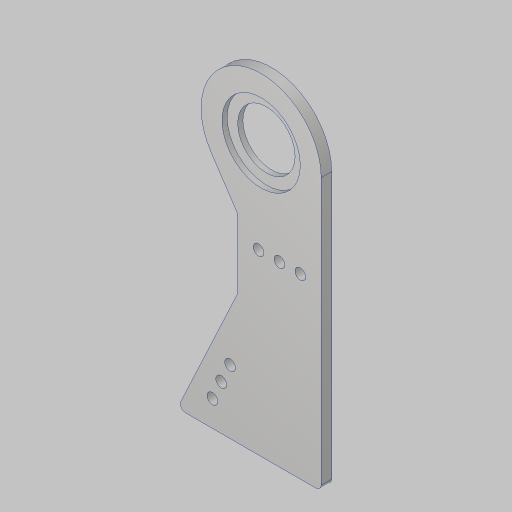
# Autodesk Inventor part: CL7-007
Saved by Autodesk Inventor 2023.5 (Build 275446000, 446)
## iProperties
Created: 2025-03-17
Part Number: CL7-007
Material: Aluminum 6061
Document SubType Name: Modeling
Designer: brand
Density: 2.7 g/cm^3
Appearance: Aluminum - Flat
Author: brand
Autodesk Inventor part; units mm, degrees
ref_plane "YZ Plane" through (0, 0, 0) normal (1, 0, 0) x (0, 1, 0)
ref_plane "XZ Plane" through (0, 0, 0) normal (0, 1, 0) x (-1, 0, 0)
ref_plane "XY Plane" through (0, 0, 0) normal (0, 0, 1) x (1, 0, 0)
sketch "Sketch1" plane through (0, 0, 0) normal (0, 0, 1) x (1, 0, 0)
  circle A0 centre (0, 0) radius 23.8125
  circle A1 centre (0, 0) radius 36.5125
  line L0 (36.5125, -165.1) -> (-14.2875, -165.1) construction
  line L1 (36.5125, 0) -> (36.5125, -165.1)
  line L2 (-36.1762, -4.9442) -> (-14.2875, -165.1) construction
  line L3 (36.5125, -44.45) -> (-14.2875, -44.45) construction
  line L4 (-14.2875, -44.45) -> (-14.2875, -431.8) construction
  line L5 (-14.2875, -431.8) -> (36.5125, -431.8) construction
  line L6 (36.5125, -431.8) -> (36.5125, -44.45) construction
  line L7 (8.7327, -97.2312) -> (-152.2848, -442.5345) construction
  line L8 (-152.2848, -442.5345) -> (-175.3051, -431.8) construction
  line L9 (-175.3051, -431.8) -> (-14.2875, -86.4967) construction
  line L10 (-14.2875, -86.4967) -> (8.7327, -97.2312) construction
  line L11 (36.5125, -431.8) -> (11.1125, -431.8) construction
  line L12 (11.1125, -431.8) -> (11.1125, -501.65) construction
  line L13 (11.1125, -501.65) -> (36.5125, -501.65) construction
  line L14 (36.5125, -501.65) -> (36.5125, -431.8) construction
  line L15 (-150.8125, -431.8) -> (-150.8125, -501.65) construction
  line L16 (-2.7774, -91.864) -> (-19.4192, -127.5524) construction
  line L17 (-36.3765, 3.1489) -> (-36.3765, -165.1) construction
  line L18 (-50.9408, -165.1) -> (36.5125, -165.1)
  line L19 (-50.9408, -165.1) -> (-36.3765, 3.1489)
  line L20 (-50.9408, -165.1) -> (-14.2875, -86.4967)
  line L21 (-14.2875, -44.45) -> (-14.2875, -86.4967)
  line L22 (-14.2875, -44.45) -> (-30.4024, -20.2202)
  point P0 (23.8125, -431.8)
  point P1 (-8.1446, -103.3741)
  point P2 (23.8125, -57.15)
  point P3 (11.1125, -57.15)
  point P4 (-1.5875, -57.15)
  point P5 (11.1125, -44.45)
  point P6 (-13.5119, -114.8842)
  point P7 (-18.8791, -126.3943)
  point P8 (-24.2464, -137.9044)
  point P9 (-29.6137, -149.4145)
  dimension "d0" = 47.625
  dimension "d1" = 12.7
  dimension "d2" = 50.8
  dimension "d3" = 165.1
  dimension "d4" = 50.8
  dimension "d5" = 387.35
  dimension "d6" = 25.4
  dimension "d7" = 25
  dimension "d8" = 381
  dimension "d10" = 25.4
  dimension "d11" = 69.85
  dimension "d13" = 431.8
  dimension "d15" = 187.325
  dimension "d17" = 12.7
  dimension "d18" = 12.7
  dimension "d19" = 12.7
  dimension "d20" = 12.7
  dimension "d23" = 12.7
  constraints: 46 end point, 6 horizontal alignment, 6 parallel, 6 point on line, 5 perpendicular, 4 tangent, 3 collinear, 3 horizontal, 3 midpoint, 3 point on circle, 2 centre point, 2 vertical, 1 coincident, 1 vertical alignment, 5 other
  measures "d0" diameter of A0
  measures "d1" radial gap between concentric circles of A0 A1
  measures "d2" distance of L0.start L0.end
  measures "d3" distance from line of L0 point (0, 0)
  measures "d4" distance of L5.end L4.end
  measures "d5" distance of L4.end L3.end
  measures "d6" distance of L7.end L8.end
  measures "d7" angle of L4 L7
  measures "d8" distance of L8.end L9.end
  measures "d10" distance of L12.end L13.end
  measures "d11" distance of L13.end L5.end
  measures "d13" vertical distance of point (23.813, -431.8) point (0, 0)
  measures "d15" distance between parallel lines of L6 L15
  measures "d17" distance of point (-8.145, -103.374) L16.start
  measures "d18" distance of point (11.113, -44.45) point (11.113, -57.15)
  measures "d19" distance of point (-1.587, -57.15) point (11.113, -57.15)
  measures "d20" distance of point (23.813, -57.15) point (11.113, -57.15)
  measures "d23" distance of point (-8.145, -103.374) point (-13.512, -114.884)
extrude "Extrusion1" add sketch "Sketch1" against normal blind 6.35 contours A1 | L1 L18 L20 L21 L22 A1
hole "Hole1" at (23.8125, -57.15, 0) at (11.1125, -57.15, 0) at (-1.5875, -57.15, 0) at (-18.8791, -126.3943, 0) at (-24.2464, -137.9044, 0) at (-29.6137, -149.4145, 0) direction (0, 0, -1) diameter 6.604 end through all
sketch "Sketch2" plane through (0, 0, -6.35) normal (0, 0, -1) x (-1, 0, 0)
  circle A0 centre (0, 0) radius 23.8125 projected
  circle A1 centre (0, 0) radius 17.4625
  dimension "d37" = 6.35
  constraints: 1 centre point
  measures "d37" radial gap between concentric circles of A0 A1
extrude "Extrusion2" add sketch "Sketch2" against normal blind 3.175
sketch "Sketch3" plane through (0, 0, 0) normal (0, 0, 1) x (1, 0, 0)
  circle A0 centre (-24.2464, -137.9044) radius 3.302 construction
  circle A1 centre (-1.5875, -57.15) radius 3.302 construction
  circle A2 centre (23.8125, -57.15) radius 3.302 construction
  circle A3 centre (11.1125, -57.15) radius 3.302 construction
  circle A4 centre (-18.8791, -126.3943) radius 3.302 construction
  circle A5 centre (-29.6137, -149.4145) radius 3.302 construction
  circle A6 centre (0, 0) radius 23.8125 construction
  line L0 (36.5125, 0) -> (36.5125, -165.1) construction
  line L1 (36.5125, -165.1) -> (-50.9408, -165.1) construction
  circle A7 centre (-24.2464, -137.9044) radius 3.302 construction
  circle A8 centre (-1.5875, -57.15) radius 3.302 construction
  circle A9 centre (23.8125, -57.15) radius 3.302 construction
  circle A10 centre (11.1125, -57.15) radius 3.302 construction
  circle A11 centre (-18.8791, -126.3943) radius 3.302 construction
  circle A12 centre (-29.6137, -149.4145) radius 3.302 construction
  circle A13 centre (0, 0) radius 23.8125 construction
  line L2 (36.5125, 0) -> (36.5125, -165.1) construction
  line L3 (36.5125, -165.1) -> (-50.9408, -165.1) construction
  line L4 (-175.3051, -431.8) -> (-14.2875, -86.4967) construction
  line L5 (8.7327, -97.2312) -> (-152.2848, -442.5345) construction
  line L6 (-14.2875, -44.45) -> (-14.2875, -431.8) construction
  line L7 (-14.2875, -86.4967) -> (-14.2875, -44.45) projected
  line L8 (-14.2875, -44.45) -> (-30.4024, -20.2202) projected
  arc A14 (36.5125, 0) -> (-30.4024, -20.2202) centre (0, 0) ccw projected
  line L9 (-50.9408, -165.1) -> (-14.2875, -86.4967) projected
  line L10 (-14.2875, -86.4967) -> (-14.2875, -44.45) projected
  line L11 (-14.2875, -44.45) -> (-30.4024, -20.2202) projected
  arc A15 (36.5125, 0) -> (-30.4024, -20.2202) centre (0, 0) ccw projected
  line L12 (-50.9408, -165.1) -> (-14.2875, -86.4967) projected
fillet "Fillet1" radius 3.175 4 edges at (-14.2875, -44.45, -3.175) (-14.2875, -86.4967, -3.175) (-50.9408, -165.1, -3.175) (36.5125, -165.1, -3.175)
equation "\"d20\" = d19"
body "Solid1"
